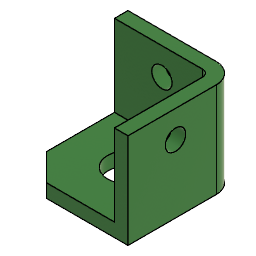
3D Bracket (Autodesk Fusion 360 archive; units mm, degrees)
design "Bracket"
part number: 2026-04-01-21-07-02-416
Autodesk Fusion 360 part; units mm, degrees
sketch "Sketch1" plane through (0, 0, 0) normal (0, 0, 1) x (1, 0, 0)
  line L0 (0, 0) -> (80, 0)
  line L1 (80, 0) -> (80, 80)
  line L2 (80, 80) -> (0, 80)
  line L3 (0, 80) -> (0, 0)
  line L4 (0, 20) -> (20, 0)
  circle A0 centre (40, 40) radius 15
  dimension "d1" = 20
  dimension "d2" = 20
  dimension "d3" = 80
  dimension "d4" = 80
  dimension "d5" = 30
  dimension "d6" = 40
  dimension "d7" = 40
  constraint horizontal L0
  constraint vertical L1
  constraint horizontal L2
  constraint vertical L3
  constraint coincident L0.start L3.end
  constraint coincident L3 L4.start
  constraint coincident L0 L4.end
  measures "d1" distance of L0.start L4.start
  measures "d2" distance of L0.start L4.end
  measures "d3" distance of L0.start L0.end
  measures "d4" distance of L0.start L2.end
  measures "d5" diameter of A0
  measures "d6" distance of L3 A0.centre
  measures "d7" distance of L0 A0.centre
extrude "Extrude1" add sketch "Sketch1" along normal blind 10 contours L0 L1 L2 L3 L4
sketch "Sketch2" plane through (0, 0, 10) normal (0, 0, 1) x (-1, 0, 0)
  circle A0 centre (-40, -40) radius 15
  line L0 (0, -20) -> (-20, 0)
  line L1 (-20, 0) -> (-80, 0)
  line L2 (-80, 0) -> (-80, -80)
  line L3 (-80, -80) -> (0, -80)
  line L4 (0, -80) -> (0, -20)
  line L5 (0, -80) -> (-80, -80)
  line L6 (-80, -80) -> (-80, -70)
  line L7 (-80, -70) -> (0, -70)
  line L8 (0, -70) -> (0, -80)
  line L9 (-70, -80) -> (-80, -80)
  line L10 (-80, -80) -> (-80, 0)
  line L11 (-80, 0) -> (-70, 0)
  line L12 (-70, 0) -> (-70, -80)
  dimension "d10" = 10
  dimension "d11" = 80
  dimension "d12" = 10
  constraint horizontal L5
  constraint vertical L6
  constraint horizontal L7
  constraint vertical L8
  constraint coincident L2 L6.end
  constraint coincident L3.end L4.start
  constraint horizontal L9
  constraint vertical L10
  constraint horizontal L11
  constraint vertical L12
  constraint coincident L1.end L2.start
  constraint coincident L5 L9.start
  measures "d10" distance of L3.end L7.end
  measures "d11" distance of L9.start L11.end
  measures "d12" distance of L1.end L11.end
extrude "Extrude2" add sketch "Sketch2" along normal blind 60 contours L3 L4 L5 L7 L8 L12 | L1 L2 L7 L10 L11 L12 | L2 L3 L5 L6 L7 L9 L10 L12
fillet "Fillet1" radius 5 1 edges at (70, 70, 40)
fillet "Fillet2" radius 15 1 edges at (80, 80, 35)
sketch "Sketch3" plane through (70, 0, 0) normal (-1, 0, 0) x (0, -1, 0)
  line L0 (-65, 70) -> (-65, 10)
  line L1 (-65, 10) -> (0, 10)
  line L2 (0, 10) -> (0, 70)
  line L3 (0, 70) -> (-65, 70)
  circle A0 centre (-35, 50) radius 7.5
  dimension "d19" = 15
  dimension "d20" = 35
  dimension "d30" = 20
  measures "d19" diameter of A0
  measures "d20" distance of L2 A0.centre
  measures "d30" distance of L3 A0.centre
extrude "Extrude3" cut sketch "Sketch3" against normal blind 10 contours A0
sketch "Sketch4" plane through (0, 70, 0) normal (0, -1, 0) x (1, 0, 0)
  line L0 (65, 10) -> (65, 70)
  line L1 (65, 70) -> (0, 70)
  line L2 (0, 70) -> (0, 10)
  line L3 (0, 10) -> (65, 10)
  circle A0 centre (35, 50) radius 7.5
  dimension "d24" = 15
  dimension "d25" = 35
  dimension "d27" = 20
  measures "d24" diameter of A0
  measures "d25" distance of L2 A0.centre
  measures "d27" distance of L1 A0.centre
extrude "Extrude4" cut sketch "Sketch4" against normal blind 50 contours A0

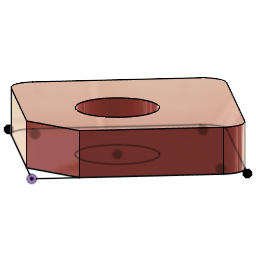
design "Baseplate"
part number: 2026-04-01-20-52-09-990
Autodesk Fusion 360 part; units mm, degrees
sketch "Sketch1" plane through (0, 0, 0) normal (0, 0, 1) x (1, 0, 0)
  line L0 (0, 0) -> (80, 0)
  line L1 (90, 10) -> (90, 80)
  line L2 (80, 90) -> (10, 90)
  line L3 (0, 80) -> (0, 0)
  line L4 (0, 20) -> (20, 0)
  circle A0 centre (40, 40) radius 17.5
  arc A1 (10, 90) -> (0, 80) centre (10, 80) ccw
  arc A2 (90, 80) -> (80, 90) centre (80, 80) ccw
  arc A3 (80, 0) -> (90, 10) centre (80, 10) ccw
  point P0 (90, 0)
  point P1 (0, 90)
  dimension "d1" = 90
  dimension "d2" = 90
  dimension "d3" = 20
  dimension "d4" = 20
  dimension "d5" = 35
  dimension "d6" = 40
  dimension "d7" = 40
  dimension "d8" = 10
  dimension "d9" = 10
  dimension "d10" = 10
  constraint horizontal L0
  constraint vertical L1
  constraint horizontal L2
  constraint vertical L3
  constraint coincident L0.start L3.end
  constraint coincident L3 L4.start
  constraint coincident L0 L4.end
  constraint coincident P1 L3
  constraint coincident P1 L2
  constraint tangent L3 A1
  constraint tangent L2 A1
  constraint tangent L2 A2
  constraint tangent L1 A2
  constraint coincident P0 L1
  constraint coincident P0 L0
  constraint tangent L1 A3
  constraint tangent L0 A3
  measures "d1" distance of L0.start P0
  measures "d2" distance of L0.start P1
  measures "d3" distance of L0.start L4.start
  measures "d4" distance of L0.start L4.end
  measures "d5" diameter of A0
  measures "d6" distance of L3 A0.centre
  measures "d7" distance of L0 A0.centre
  measures "d8" radius of A1
  measures "d9" radius of A2
  measures "d10" radius of A3
extrude "Extrude1" add sketch "Sketch1" along normal blind 10 contours L0 L1 L2 L3 L4 A1 A2 A3
extrude "Extrude2" add 1 faces at (79.1015, 44.2027, 10) along direction (0, 0, 1) blind 10

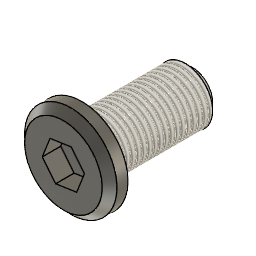
design "Fastner"
part number: 2026-04-01-21-23-47-223
Autodesk Fusion 360 part; units mm, degrees
sketch "Sketch1" plane through (0, 0, 0) normal (0, 1, 0) x (1, 0, 0)
  circle A0 centre (0, 0) radius 7.5
  dimension "d1" = 15
  constraint coincident A0.centre origin
  measures "d1" diameter of A0
extrude "Extrude1" add sketch "Sketch1" along normal blind 30
sketch "Sketch2" plane through (0, 0, 0) normal (0, -1, 0) x (1, 0, 0)
  circle A0 centre (0, 0) radius 7.5
  circle A1 centre (0, 0) radius 12.5
  dimension "d4" = 25
  constraint coincident A0.centre A1.centre
  measures "d4" diameter of A1
extrude "Extrude2" add sketch "Sketch2" along normal blind 5 contours A0 | A1
chamfer "Chamfer1" distance 2 angle 45 2 edges at (-11.6541, -5, -4.5202) (-6.9925, 30, 2.7121)
thread "Thread1" "ISO Metric profile 15.0 M15x1.5 M15x1.5 6g" major diameter 14.85 minor diameter 13.1369 pitch 1.5 angle 60 resizes the face on face at (7.4907, 18.6667, 0.3738)
sketch "Sketch3" plane through (0, -5, 0) normal (0, -1, 0) x (1, 0, 0)
  circle A0 centre (0, 0) radius 10.5
  line L0 (2.101, 5.3776) -> (-3.6067, 4.5083)
  line L1 (-3.6067, 4.5083) -> (-5.7077, -0.8693)
  line L2 (-5.7077, -0.8693) -> (-2.101, -5.3776)
  line L3 (-2.101, -5.3776) -> (3.6067, -4.5083)
  line L4 (3.6067, -4.5083) -> (5.7077, 0.8693)
  line L5 (5.7077, 0.8693) -> (2.101, 5.3776)
  dimension "d10" = 5
  constraint coincident A0.centre origin
  measures "d10" distance of A0.centre L5
extrude "Extrude3" cut sketch "Sketch3" against normal blind 5 contours L0 L1 L2 L3 L4 L5
